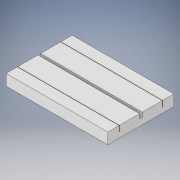
# Autodesk Inventor part: Small Bread Board
Saved by Autodesk Inventor 2018 (Build 220112000, 112)
## iProperties
Created: 2018-05-02
Part Number: Small Bread Board
Material: PC/ABS Plastic
Document SubType Name: Modeling
Designer: Ajith Thomas
Density: 0.357273 g/cm^3
Appearance: Smooth - White
Mass: 14.1242 g
Surface Area: 135.488 cm^2
Volume: 39.5335 cm^3
Author: Ajith Thomas
Autodesk Inventor part; units mm, degrees
ref_plane "YZ Plane" through (0, 0, 0) normal (1, 0, 0) x (0, 1, 0)
ref_plane "XZ Plane" through (0, 0, 0) normal (0, 1, 0) x (-1, 0, 0)
ref_plane "XY Plane" through (0, 0, 0) normal (0, 0, 1) x (1, 0, 0)
sketch "Sketch1" plane through (0, 0, 0) normal (0, 1, 0) x (-1, 0, 0)
  line L0 (41.5, -27) -> (-41.5, -27)
  line L1 (-41.5, -27) -> (-41.5, 27)
  line L2 (-41.5, 27) -> (41.5, 27)
  line L3 (41.5, 27) -> (41.5, -27)
  line L4 (41.5, -27) -> (-41.5, 27) construction
  line L5 (-41.5, -27) -> (41.5, 27) construction
  point P0 (0, 0)
  dimension "d0" = 83
  dimension "d1" = 54
  constraints: 12 end point, 2 midpoint, 2 parallel, 1 horizontal, 1 perpendicular
  measures "d0" distance of L1.end L2.end
  measures "d1" distance of L0.end L1.end
extrude "Extrusion1" add sketch "Sketch1" along normal blind 9
sketch "Sketch2" plane through (41.5, 0, 27) normal (1, 0, 0) x (0, 0, -1)
  line L0 (27, 0) -> (27, 8.8182) construction
  line L1 (27, 4.4091) -> (44.5, 4.4091) construction
  line L2 (44.5, 4.4091) -> (44.75, 4.4091)
  line L3 (44.75, 4.4091) -> (44.75, 11.998)
  line L4 (44.75, 11.998) -> (44.5, 11.998)
  line L5 (44.5, 11.998) -> (44.5, 4.4091)
  line L6 (9.5, 4.4091) -> (9.25, 4.4091)
  line L7 (9.25, 4.4091) -> (9.25, 11.998)
  line L8 (9.25, 11.998) -> (9.5, 11.998)
  line L9 (9.5, 11.998) -> (9.5, 4.4091)
  line L10 (26, 12.3352) -> (28, 12.3352)
  line L11 (28, 12.3352) -> (28, 5.3012)
  line L12 (28, 5.3012) -> (26, 5.3012)
  line L13 (26, 5.3012) -> (26, 12.3352)
  line L14 (26, 12.3352) -> (28, 5.3012) construction
  line L15 (28, 12.3352) -> (26, 5.3012) construction
  dimension "d4" = 17.5
  dimension "d5" = 0.25
  dimension "d6" = 2
  dimension "d7" = 7.034
  constraints: 32 end point, 4 parallel, 4 symmetric about line, 3 horizontal, 3 midpoint, 2 perpendicular, 1 vertical
  measures "d4" distance of L1.start L1.end
  measures "d5" distance of L4.end L3.end
  measures "d6" distance of L11.end L12.end
  measures "d7" distance of L10.end L11.end
extrude "Extrusion2" cut sketch "Sketch2" against normal blind 109.0125
body "Solid1"
